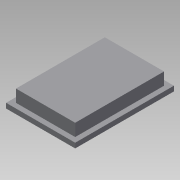
# Autodesk Inventor part: User Control Panel - Rough
Saved by Autodesk Inventor 2015 (Build 190159000, 159)
## iProperties
Created: 2015-05-21
Part Number: User Control Panel - Rough
Material: Generic
Document SubType Name: Modeling
Designer: Joe Sheldon
Density: 1 g/cm^3
Appearance: Default
Author: Joe Sheldon
Autodesk Inventor part; units mm, degrees
ref_plane "YZ Plane" through (0, 0, 0) normal (1, 0, 0) x (0, 1, 0)
ref_plane "XZ Plane" through (0, 0, 0) normal (0, 1, 0) x (-1, 0, 0)
ref_plane "XY Plane" through (0, 0, 0) normal (0, 0, 1) x (1, 0, 0)
sketch "Sketch1" plane through (0, 0, 0) normal (0, 1, 0) x (-1, 0, 0)
  line L0 (-38.1, 57.15) -> (38.1, 57.15)
  line L1 (38.1, 57.15) -> (38.1, -57.15)
  line L2 (38.1, -57.15) -> (-38.1, -57.15)
  line L3 (-38.1, -57.15) -> (-38.1, 57.15)
  line L4 (-38.1, 57.15) -> (38.1, -57.15) construction
  line L5 (38.1, 57.15) -> (-38.1, -57.15) construction
  line L6 (44.45, -63.5) -> (44.45, 63.5)
  line L7 (44.45, 63.5) -> (-44.45, 63.5)
  line L8 (-44.45, 63.5) -> (-44.45, -63.5)
  line L9 (-44.45, -63.5) -> (44.45, -63.5)
  point P0 (0, 0)
  dimension "d0" = 76.2
  dimension "d1" = 114.3
  dimension "d2" = 6.35
  constraints: 20 end point, 4 parallel, 2 midpoint, 2 perpendicular, 1 horizontal, 3 other
  measures "d0" distance of L1.end L2.end
  measures "d1" distance of L0.end L1.end
  measures "d2" distance between parallel lines of L1 L6
extrude "Extrusion1" add sketch "Sketch1" along normal blind 6.35
sketch "Sketch2" plane through (0, 6.35, 0) normal (0, 1, 0) x (1, 0, 0)
  line L0 (-38.1, -57.15) -> (-38.1, 57.15) projected
  line L1 (-38.1, 57.15) -> (38.1, 57.15) projected
  line L2 (38.1, 57.15) -> (38.1, -57.15) projected
  line L3 (38.1, -57.15) -> (-38.1, -57.15) projected
  line L4 (-44.45, 63.5) -> (-44.45, -63.5) projected
  line L5 (-44.45, -63.5) -> (44.45, -63.5) projected
  line L6 (44.45, -63.5) -> (44.45, 63.5) projected
  line L7 (44.45, 63.5) -> (-44.45, 63.5) projected
  point P0 (0, 0)
extrude "Extrusion2" add sketch "Sketch2" along normal mid plane 6.35 contours L0 L1 L2 L3
sketch "Sketch3" plane through (0, 9.525, 0) normal (0, 1, 0) x (1, 0, 0)
  line L0 (-38.1, 57.15) -> (-38.1, -57.15) projected
  line L1 (-38.1, -57.15) -> (38.1, -57.15) projected
  line L2 (38.1, -57.15) -> (38.1, 57.15) projected
  line L3 (38.1, 57.15) -> (-38.1, 57.15) projected
  point P0 (0, 0)
extrude "Extrusion3" add sketch "Sketch3" along normal blind 12.7
body "Solid1"
